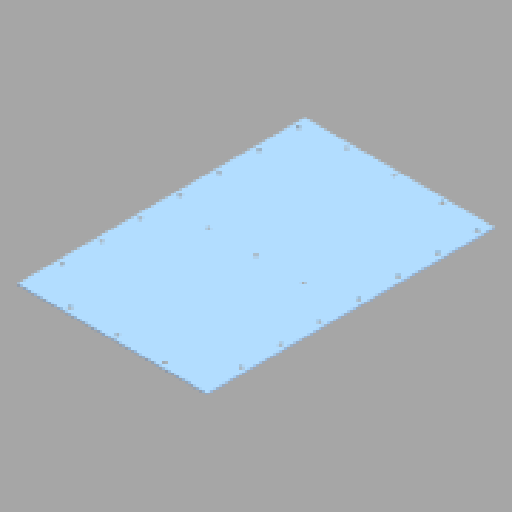
# Autodesk Inventor part: нижняя плита
Saved by Autodesk Inventor 2025 (Build 290162000, 162)
## iProperties
Created: 2025-01-21
Part Number: нижняя плита
Material: СВМПЭ, белый
Document SubType Name: Modeling
Designer: volko
Density: 0.94 g/cm^3
Appearance: Гладкий — белый
Mass: 840.848 g
Surface Area: 3697.01 cm^2
Volume: 894.519 cm^3
Author: volko
Autodesk Inventor part; units mm, degrees
ref_plane "YZ Plane" through (0, 0, 0) normal (1, 0, 0) x (0, 1, 0)
ref_plane "XZ Plane" through (0, 0, 0) normal (0, 1, 0) x (-1, 0, 0)
ref_plane "XY Plane" through (0, 0, 0) normal (0, 0, 1) x (1, 0, 0)
sketch "Эскиз1" plane through (0, 0, 0) normal (0, 1, 0) x (-1, 0, 0)
  line L0 (0, 265) -> (175, 265)
  line L1 (175, 265) -> (175, -265)
  line L2 (0, 265) -> (0, 0)
  line L3 (0, 0) -> (200, 0)
  line L4 (0, 265) -> (-175, 265)
  line L5 (-175, 265) -> (-175, -265)
  line L6 (0, -265) -> (175, -265)
  line L7 (175, -265) -> (175, -125)
  line L8 (-175, -265) -> (-175, -125)
  line L9 (0, -265) -> (-175, -265)
  point P0 (175, 125)
  point P1 (-175, 125)
  dimension "d3" = 350
  dimension "d6" = 530
  constraints: 20 end point, 7 symmetric about line, 4 point on line, 1 vertical
  measures "d3" distance between parallel lines of L5 L1
  measures "d6" distance between parallel lines of L4 L9
extrude "Выдавливание1" add sketch "Эскиз1" along normal blind 2
sketch "Эскиз2" plane through (0, 0, 0) normal (0, 1, 0) x (1, 0, 0)
  line L0 (-175, -265) -> (175, -265) projected
  line L1 (175, -265) -> (175, 265) projected
  point P0 (0, 0)
  point P1 (87.5, -255)
  point P2 (0, -255)
  point P3 (-87.5, -255)
  point P4 (87.5, 0)
  point P5 (0, 0)
  point P6 (-87.5, 0)
  point P7 (87.5, 255)
  point P8 (0, 255)
  point P9 (-87.5, 255)
  point P10 (165, -198.75)
  point P11 (165, -132.5)
  point P12 (165, -66.25)
  point P13 (165, 0)
  point P14 (165, 66.25)
  point P15 (165, 132.5)
  point P16 (165, 198.75)
  point P17 (-165, -198.75)
  point P18 (-165, -132.5)
  point P19 (-165, -66.25)
  point P20 (-165, 0)
  point P21 (-165, 66.25)
  point P22 (-165, 132.5)
  point P23 (-165, 198.75)
  dimension "d15" = 10
  dimension "d16" = 87.5
  dimension "d19" = 87.5
  dimension "d22" = 255
  dimension "d25" = 10
  dimension "d26" = 66.25
  dimension "d29" = 66.25
  dimension "d32" = 330
  constraints: 2 horizontal, 2 vertical, 21 other
  measures "d15" distance from line of L0 point (87.5, -255)
  measures "d16" distance from line of point (87.5, -255) L1
  measures "d19" distance of point (87.5, -255) point (0, -255)
  measures "d22" distance of point (87.5, -255) point (87.5, 0)
  measures "d25" distance from line of point (165, -198.75) L1
  measures "d26" distance from line of L0 point (165, -198.75)
  measures "d29" distance of point (165, -198.75) point (165, -132.5)
  measures "d32" distance of point (165, -198.75) point (-165, -198.75)
hole "Отверстие2" at (87.5, 0, 255) at (0, 0, 255) at (-87.5, 0, 255) at (87.5, 0, 0) at (0, 0, 0) at (-87.5, 0, 0) at (87.5, 0, -255) at (0, 0, -255) at (-87.5, 0, -255) at (165, 0, 198.75) at (165, 0, 132.5) at (165, 0, 66.25) at (165, 0, 0) at (165, 0, -66.25) at (165, 0, -132.5) at (165, 0, -198.75) at (-165, 0, 198.75) at (-165, 0, 132.5) at (-165, 0, 66.25) at (-165, 0, 0) at (-165, 0, -66.25) at (-165, 0, -132.5) at (-165, 0, -198.75) direction (0, 1, 0) diameter 3 end through all countersink diameter 11 countersink angle 90
sketch "Эскиз3" plane through (0, 0, 0) normal (0, -1, 0) x (1, 0, 0)
  line L0 (-245, 0) -> (245, 0) projected
  line L1 (0, -371) -> (0, 371) projected
  line L2 (-175, 265) -> (175, 265) projected
  point P0 (0, 0)
  point P1 (120, 207)
  point P2 (64, 207)
  point P3 (120, 235)
  point P4 (64, 235)
  point P5 (-120, 207)
  point P6 (-64, 207)
  point P7 (-120, 235)
  point P8 (-64, 235)
  point P9 (120, -207)
  point P10 (64, -207)
  point P11 (120, -235)
  point P12 (64, -235)
  point P13 (-120, -235)
  point P14 (-120, -207)
  point P15 (-64, -207)
  point P16 (-64, -235)
  dimension "d52" = 56
  dimension "d55" = 28
  dimension "d59" = 120
  dimension "d60" = 30
  constraints: 12 symmetric about line, 1 horizontal, 1 vertical, 3 other
  measures "d52" distance of point (120, 207) point (64, 207)
  measures "d55" distance of point (120, 207) point (120, 235)
  measures "d59" distance from line of L1 point (120, 207)
  measures "d60" distance from line of L2 point (120, 235)
